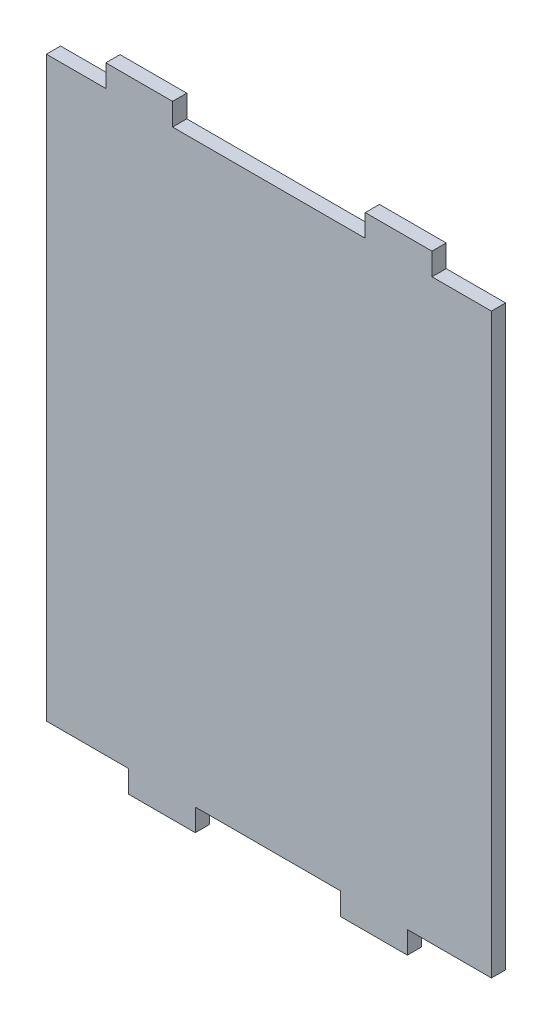
# Autodesk Inventor part: SideWall_new
Saved by Autodesk Inventor 2017 (Build 210142000, 142)
## iProperties
Created: 2017-05-28
Part Number: SideWall_new
Material: Generic
Document SubType Name: Modeling
Designer: Paolo
Density: 1 g/cm^3
Appearance: Default
Author: Paolo
Autodesk Inventor part; units mm, degrees
ref_plane "YZ Plane" through (0, 0, 0) normal (1, 0, 0) x (0, 1, 0)
ref_plane "XZ Plane" through (0, 0, 0) normal (0, 1, 0) x (-1, 0, 0)
ref_plane "XY Plane" through (0, 0, 0) normal (0, 0, 1) x (1, 0, 0)
sketch "NewProfile" plane through (0, 0, 0) normal (0, 0, 1) x (1, 0, 0)
  line L0 (28.6811, -6) -> (28.8811, -4) projected
  line L1 (44.2811, -6) -> (28.6811, -6) projected
  line L2 (44.0811, -4) -> (44.2811, -6) projected
  line L3 (28.8811, -4) -> (44.0811, -4) projected
  line L4 (-10.7189, -4) -> (-10.5189, -6) projected
  line L5 (-25.9189, -4) -> (-10.7189, -4) projected
  line L6 (-26.1189, -6) -> (-25.9189, -4) projected
  line L7 (-10.5189, -6) -> (-26.1189, -6) projected
  line L8 (44.2811, -128) -> (44.0811, -130) projected
  line L9 (28.6811, -128) -> (44.2811, -128) projected
  line L10 (28.8811, -130) -> (28.6811, -128) projected
  line L11 (44.0811, -130) -> (28.8811, -130) projected
  line L12 (-26.1189, -128) -> (-25.9189, -130) projected
  line L13 (-10.7189, -130) -> (-25.9189, -130) projected
  line L14 (-10.5189, -128) -> (-10.7189, -130) projected
  line L15 (-26.1189, -128) -> (-10.5189, -128) projected
  line L16 (-37.9189, -6) -> (56.0811, -6)
  line L17 (56.0811, -6) -> (56.0811, -128)
  line L18 (56.0811, -128) -> (-37.9189, -128)
  line L19 (-37.9189, -128) -> (-37.9189, -6)
  line L20 (-25.3689, -6) -> (-11.2689, -6)
  line L21 (-11.2689, -6) -> (-11.2689, -1.3)
  line L22 (-11.2689, -1.3) -> (-25.3689, -1.3)
  line L23 (-25.3689, -1.3) -> (-25.3689, -6)
  line L24 (29.4311, -6) -> (43.5311, -6)
  line L25 (43.5311, -6) -> (43.5311, -1.3)
  line L26 (43.5311, -1.3) -> (29.4311, -1.3)
  line L27 (29.4311, -1.3) -> (29.4311, -6)
  line L28 (-26.1189, -128) -> (-26.1189, -6) construction
  line L29 (-21.1189, -128) -> (-20.9189, -130) construction
  line L30 (-5.7189, -130) -> (-20.9189, -130) construction
  line L31 (-5.7189, -130) -> (-5.5189, -128) construction
  line L32 (-21.1189, -128) -> (-5.5189, -128) construction
  line L33 (39.0811, -130) -> (39.2811, -128) construction
  line L34 (23.6811, -128) -> (39.2811, -128) construction
  line L35 (23.8811, -130) -> (23.6811, -128) construction
  line L36 (39.0811, -130) -> (23.8811, -130) construction
  line L37 (-21.1189, -128) -> (-21.1189, -6) construction
  line L38 (-21.1189, -128) -> (100.8811, -128) construction
  line L39 (-10.5189, -128) -> (-10.5189, -6) construction
  line L40 (-10.5189, -128) -> (111.4811, -128) construction
  line L41 (-5.5189, -128) -> (-5.5189, -6) construction
  line L42 (-5.5189, -128) -> (116.4811, -128) construction
  line L43 (23.6811, -128) -> (23.6811, -6) construction
  line L44 (28.6811, -128) -> (28.6811, -6) construction
  line L45 (39.2811, -128) -> (39.2811, -6) construction
  line L46 (44.2811, -128) -> (44.2811, -6) construction
  line L47 (-5.5189, -6) -> (-5.7189, -4) construction
  line L48 (-20.9189, -4) -> (-5.7189, -4) construction
  line L49 (-20.9189, -4) -> (-21.1189, -6) construction
  line L50 (-5.5189, -6) -> (-21.1189, -6) construction
  line L51 (39.2811, -6) -> (39.0811, -4) construction
  line L52 (23.8811, -4) -> (39.0811, -4) construction
  line L53 (23.8811, -4) -> (23.6811, -6) construction
  line L54 (39.2811, -6) -> (23.6811, -6) construction
  line L55 (-20.5689, -128) -> (-6.4689, -128)
  line L56 (-6.4689, -128) -> (-6.4689, -132.7)
  line L57 (-6.4689, -132.7) -> (-20.5689, -132.7)
  line L58 (-20.5689, -132.7) -> (-20.5689, -128)
  line L59 (24.2311, -128) -> (38.3311, -128)
  line L60 (38.3311, -128) -> (38.3311, -132.7)
  line L61 (38.3311, -132.7) -> (24.2311, -132.7)
  line L62 (24.2311, -132.7) -> (24.2311, -128)
  point P0 (0, 0)
  dimension "d0" = 94
  dimension "d1" = 122
  dimension "d2" = 11.8
  dimension "d3" = 11.8
  dimension "d4" = 14.1
  dimension "d5" = 4.7
  dimension "d6" = 14.1
  dimension "d7" = 4.7
  dimension "d21" = 0.55
  dimension "d23" = 15.2
  dimension "d24" = 15.2
  dimension "d25" = 0.55
  dimension "d26" = 14.1
  dimension "d27" = 4.7
  dimension "d28" = 14.1
  dimension "d29" = 4.7
  dimension "d30" = 15.2
  dimension "d31" = 0.55
  dimension "d32" = 0.55
  dimension "d33" = 15.2
  constraints: 62 end point, 11 parallel, 11 perpendicular, 8 horizontal, 6 point on line, 2 vertical, 1 collinear
  measures "d0" distance of L16.start L16.end
  measures "d1" distance between parallel lines of L18 L16
  measures "d2" distance from line of L19 L6.start
  measures "d3" distance from line of L1.start L17
  measures "d4" distance of L22.end L21.end
  measures "d5" distance of L21.end L20.end
  measures "d6" distance of L26.end L25.end
  measures "d7" distance of L25.end L24.end
  measures "d21" distance from line of L5.start L23
  measures "d23" distance of L5.start L4.start
  measures "d24" distance of L0.end L2.start
  measures "d25" distance from line of L0.end L27
  measures "d26" distance of L56.end L57.end
  measures "d27" distance of L55.end L56.end
  measures "d28" distance of L60.end L61.end
  measures "d29" distance of L59.end L60.end
  measures "d30" distance of L30.start L29.end
  measures "d31" distance of L29.start L55.start
  measures "d32" distance from line of L34.start L62
  measures "d33" distance of L8.end L10.start
extrude "Extrusion1" add sketch "NewProfile" against normal blind 3 contours L1 L16 L17 L18 L9 L15 L19 L7 | L27 L3 L25 L1 | L27 L26 L25 L3 | L7 L23 L5 L21 | L5 L23 L22 L21 | L60 L11 L10 L9 | L60 L61 L62 L18 L10 L11 | L15 L14 L13 L58 | L13 L14 L18 L56 L57 L58
equation "\"d21\" = -0.5 * d4 + 0.5 * d23"
equation "\"d25\" = -0.5 * d6 + 0.5 * d24"
equation "\"d31\" = -0.5 * d26 + 0.5 * d30"
equation "\"d32\" = -0.5 * d28 + 0.5 * d33"
body "Solid1"
